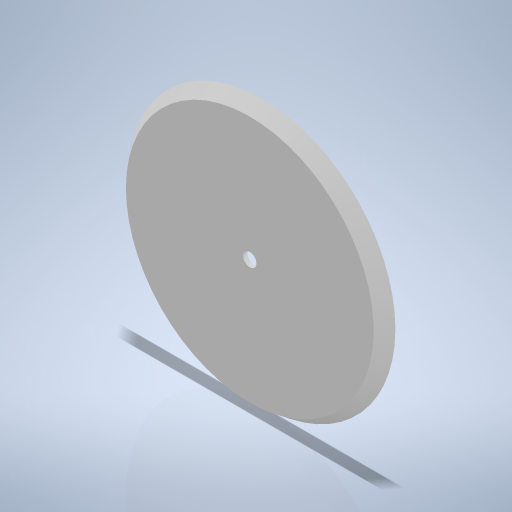
# Autodesk Inventor part: mesh filter
Saved by Autodesk Inventor 2024 (Build 280153000, 153)
## iProperties
Created: 2024-04-24
Part Number: mesh filter
Material: Generisch
Document SubType Name: Modeling
Designer: ffogue
Density: 1 g/cm^3
Appearance: Vorgabe
Author: ffogue
Autodesk Inventor part; units mm, degrees
ref_plane "YZ Plane" through (0, 0, 0) normal (1, 0, 0) x (0, 1, 0)
ref_plane "XZ Plane" through (0, 0, 0) normal (0, 1, 0) x (-1, 0, 0)
ref_plane "XY Plane" through (0, 0, 0) normal (0, 0, 1) x (1, 0, 0)
sketch "Skizze1" plane through (0, 0, 0) normal (0, 0, 1) x (1, 0, 0)
  line L0 (0, 0) -> (0, 16.3048)
  line L1 (0, 0) -> (14.75, 0)
  line L2 (14.75, 0) -> (15.5, 1)
  line L3 (15.5, 1) -> (0, 1)
  dimension "d1" = 31
  dimension "d2" = 29.5
  dimension "d3" = 1
  constraints: 8 end point, 1 horizontal, 1 parallel, 1 point on line, 1 vertical
  measures "d1" diameter of L2.end L0
  measures "d2" diameter of L1.end L0
  measures "d3" distance from line of L1 L2.end
revolve "Umdrehung1" add sketch "Skizze1" angle 360 about axis through (0, 0, 0) along (0, 1, 0)
shell "Wandung1" thickness 0.5 outward yes removed faces 1 at (2.935, 1, -4.2521)
sketch "Skizze2" plane through (0, 0, 0) normal (0, 1, 0) x (1, 0, 0)
  circle A0 centre (0, 0) radius 0.81
  dimension "d5" = 1.62
  constraints: 1 centre point, 1 coincident
  measures "d5" diameter of A0
extrude "Extrusion1" cut sketch "Skizze2" against normal up to surface (0.5 mm away)
